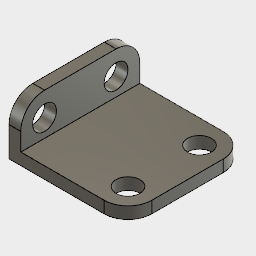
Challenge3_CSA011010 (Autodesk Fusion 360 design; units mm, degrees)
Autodesk Fusion 360 part; units mm, degrees
sketch "Sketch1" plane through (0, 0, 0) normal (0, 0, 1) x (1, 0, 0)
  line L0 (0, 0) -> (0, 45)
  line L1 (0, 45) -> (10, 45)
  line L2 (10, 45) -> (10, 10)
  line L3 (10, 10) -> (100, 10)
  line L4 (100, 10) -> (100, 0)
  line L5 (100, 0) -> (0, 0)
  dimension "d1" = 10
  dimension "d2" = 100
  dimension "d3" = 45
  measures "d1" distance of L0.end L1.end
  measures "d2" distance of L4.end L0.start
  measures "d3" distance of L0.start L0.end
extrude "Extrude1" add sketch "Sketch1" along normal mid plane 100
fillet "Fillet1" radius 20 4 edges at (5, 45, 50) (5, 45, -50) (100, 5, -50) (100, 5, 50)
sketch "Sketch2" plane through (10, 0, 0) normal (1, 0, 0) x (0, 0, -1)
  arc A0 (50, 25) -> (30, 45) centre (30, 25) ccw
  line L0 (30, 45) -> (-30, 45)
  arc A1 (-30, 45) -> (-50, 25) centre (-30, 25) ccw
  line L1 (-50, 25) -> (-50, 10)
  line L2 (-50, 10) -> (50, 10)
  line L3 (50, 10) -> (50, 25)
  circle A2 centre (-30, 25) radius 10
  circle A3 centre (30, 25) radius 10
  dimension "d7" = 20
  measures "d7" diameter of A2
extrude "Extrude2" cut sketch "Sketch2" against normal through all contours A2 | A3
sketch "Sketch3" plane through (0, 10, 0) normal (0, 1, 0) x (-1, 0, 0)
  arc A0 (-80, 50) -> (-100, 30) centre (-80, 30) ccw
  line L0 (-100, 30) -> (-100, -30)
  arc A1 (-100, -30) -> (-80, -50) centre (-80, -30) ccw
  line L1 (-80, -50) -> (-10, -50)
  line L2 (-10, -50) -> (-10, 50)
  line L3 (-10, 50) -> (-80, 50)
  circle A2 centre (-80, -30) radius 10
  circle A3 centre (-80, 30) radius 10
  dimension "d9" = 20
  measures "d9" diameter of A2
extrude "Extrude3" cut sketch "Sketch3" against normal through all contours A2 | A3
